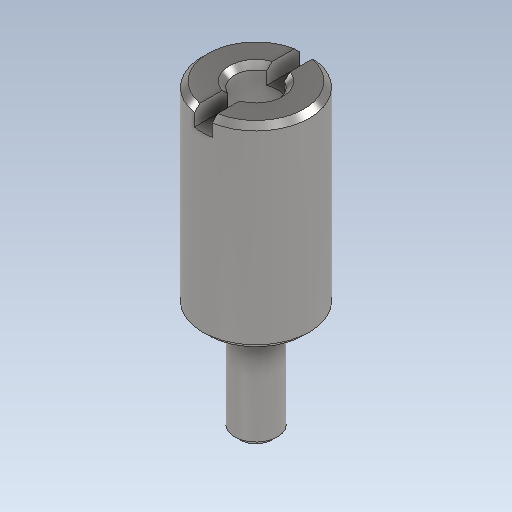
# Autodesk Inventor part: BRU-311S
Saved by Autodesk Inventor 2020.4 (Build 244396000, 396)
## iProperties
Created: 2021-09-06
Part Number: BRU-311S
Material: ステンレス鋼 AISI 304
Document SubType Name: Modeling
Designer: Masato
Density: 8 g/cm^3
Appearance: 半つや出し
Mass: 2.22137 g
Surface Area: 2.98647 cm^2
Volume: 0.277671 cm^3
Author: Masato Kubotera
Autodesk Inventor part; units mm, degrees
ref_plane "YZ Plane" through (0, 0, 0) normal (1, 0, 0) x (0, 1, 0)
ref_plane "XZ Plane" through (0, 0, 0) normal (0, 1, 0) x (-1, 0, 0)
ref_plane "XY Plane" through (0, 0, 0) normal (0, 0, 1) x (1, 0, 0)
sketch "スケッチ1" plane through (0, 0, 0) normal (0, 0, 1) x (1, 0, 0)
  line L0 (0, -7) -> (0.9, -7)
  line L1 (0.9, -7) -> (1.2, -6.7)
  line L2 (1.2, -6.7) -> (1.2, -1.5)
  line L3 (1.2, -1.5) -> (1.5, -1.5)
  line L4 (1.5, -1.5) -> (1.5, -1)
  line L5 (1.5, -1) -> (2.7, -1)
  line L6 (3, 9.7) -> (2.7, 10)
  line L7 (2.7, 10) -> (1.5, 10)
  line L8 (1.5, 10) -> (1.2, 9.7)
  line L9 (0, 7.4044) -> (0, -7.4044) construction
  line L10 (0, -7) -> (0, 7)
  line L11 (0, 7) -> (1.2, 7)
  line L12 (1.2, 7) -> (1.2, 9.7)
  line L13 (2.7, -1) -> (3, -0.7)
  line L14 (3, -0.7) -> (3, 9.7)
  point P0 (0, 0)
  point P1 (0, 0)
  point P2 (0, 0)
  dimension "d0" = 2.4
  dimension "d1" = 6
  dimension "d2" = 0.3
  dimension "d3" = 0.3
  dimension "d4" = 3
  dimension "d5" = 0.5
  dimension "d6" = 11
  dimension "d7" = 0.3
  dimension "d8" = 2.4
  dimension "d9" = 3
  dimension "d10" = 0.3
  dimension "d11" = 0.3
  dimension "d12" = 0.3
  dimension "d13" = 0.3
  dimension "d14" = 6
  constraints: 30 end point, 4 perpendicular, 4 vertical, 2 coincident, 2 horizontal, 2 midpoint, 1 collinear, 1 parallel
  measures "d0" diameter of L2 L9
  measures "d1" distance between parallel lines of L0 L5
  measures "d2" distance from line of L2.start L0
  measures "d3" horizontal distance of L2.start L1.start
  measures "d4" diameter of L4 L9
  measures "d5" distance of L3.end L5.start
  measures "d6" distance between parallel lines of L7 L5
  measures "d7" horizontal distance of L8.start L12.end
  measures "d8" diameter of L12 L9
  measures "d9" distance between parallel lines of L11 L7
  measures "d10" horizontal distance of L14.end L7.start
  measures "d11" horizontal distance of L14.end L7.start
  measures "d12" distance from line of L13.end L5
  measures "d13" horizontal distance of L5.end L13.end
  measures "d14" diameter of L14 L9
revolve "回転1" add sketch "スケッチ1" angle 360 about axis through (0, 7.4044, 0) along (0, -1, 0)
sketch "スケッチ2" plane through (0, 10, 0) normal (0, 1, 0) x (1, 0, 0)
  line L0 (-0.5, 3) -> (0.5, 3)
  line L1 (0.5, 3) -> (0.5, -3)
  line L2 (0.5, -3) -> (-0.5, -3)
  line L3 (-0.5, -3) -> (-0.5, 3)
  line L4 (-0.5, 3) -> (0.5, -3) construction
  line L5 (0.5, 3) -> (-0.5, -3) construction
  circle A0 centre (0, 0) radius 3 projected
  point P0 (0, 0)
  point P1 (0.5, 2.958)
  point P2 (-0.5, 2.958)
  point P3 (-0.5, -2.958)
  point P4 (0.5, -2.958)
  dimension "d16" = 1
  constraints: 12 end point, 2 midpoint, 2 parallel, 1 horizontal, 1 perpendicular, 1 tangent
  measures "d16" distance of L1.end L2.end
extrude "押し出し1" cut sketch "スケッチ2" against normal blind 1 contours A0 L1 L3
equation "\"d3\" = d2"
equation "\"d10\" = d7"
equation "\"d11\" = d7"
equation "\"d12\" = d11"
equation "\"d13\" = d12"
